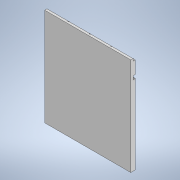
# Autodesk Inventor part: wall
Saved by Autodesk Inventor 2022 (Build 260153000, 153)
## iProperties
Created: 2022-02-20
Part Number: wall
Material: Generic
Document SubType Name: Modeling
Designer: MarkP
Density: 1 g/cm^3
Appearance: Default
Author: MarkP
Autodesk Inventor part; units mm, degrees
ref_plane "YZ Plane" through (0, 0, 0) normal (1, 0, 0) x (0, 1, 0)
ref_plane "XZ Plane" through (0, 0, 0) normal (0, 1, 0) x (-1, 0, 0)
ref_plane "XY Plane" through (0, 0, 0) normal (0, 0, 1) x (1, 0, 0)
sketch "Sketch1" plane through (0, 0, 0) normal (0, 0, 1) x (1, 0, 0)
  line L0 (0, 0) -> (750, 0)
  line L1 (750, 0) -> (750, 850)
  line L2 (750, 850) -> (0, 850)
  line L3 (0, 850) -> (0, 0)
  dimension "d0" = 750
  dimension "d1" = 850
  constraints: 8 end point, 2 parallel, 1 horizontal, 1 perpendicular
  measures "d0" distance of L2.end L1.end
  measures "d1" distance of L1.end L0.end
extrude "Extrusion1" add sketch "Sketch1" along normal blind 40
sketch "Sketch2" plane through (0, 850, 0) normal (0, 1, 0) x (1, 0, 0)
  line L0 (750, 0) -> (0, 0) projected
  line L1 (0, 0) -> (750, 0)
  line L2 (750, 0) -> (750, -20)
  line L3 (750, -20) -> (0, -20)
  line L4 (0, -20) -> (0, 0)
  dimension "d4" = 750
  dimension "d5" = 20
  constraints: 8 end point, 2 parallel, 1 horizontal, 1 perpendicular
  measures "d4" distance of L2.end L3.end
  measures "d5" distance of L1.end L2.end
extrude "Extrusion2" cut sketch "Sketch2" against normal blind 20
sketch "Sketch3" plane through (0, 850, 40) normal (0, 1, 0) x (1, 0, 0)
  line L0 (0, 20) -> (0, 0) projected
  circle A0 centre (562, 20) radius 5
  circle A1 centre (375, 20) radius 5
  circle A2 centre (188, 20) radius 5
  point P0 (0, 40)
  dimension "d11" = 10
  dimension "d12" = 10
  dimension "d13" = 10
  constraints: 3 centre point
  measures "d11" diameter of A0
  measures "d12" diameter of A1
  measures "d13" diameter of A2
extrude "Extrusion3" cut sketch "Sketch3" against normal blind 40
thread "Thread1" size "M10x1.5" class "6H" standard "ANSI Metric M Profile" full length
thread "Thread2" size "M10x1.5" class "6H" standard "ANSI Metric M Profile" full length
thread "Thread3" size "M10x1.5" class "6H" standard "ANSI Metric M Profile" full length
sketch "Sketch4" plane through (0, 0, 0) normal (0, 0, -1) x (-1, 0, 0)
  line L0 (-750, 720) -> (0, 720)
  line L1 (0, 850) -> (0, 0) projected
  line L2 (-750, 720) -> (0, 720)
  line L3 (0, 720) -> (0, 690)
  line L4 (0, 690) -> (-750, 690)
  line L5 (-750, 690) -> (-750, 720)
  line L6 (0, 690) -> (-420, 690)
  line L7 (-420, 690) -> (-420, 720)
  line L8 (-420, 720) -> (0, 720)
  line L9 (0, 720) -> (0, 690)
  dimension "d23" = 30
  dimension "d24" = 420
  dimension "d25" = 30
  constraints: 18 end point, 4 parallel, 2 horizontal, 2 perpendicular, 1 point on line
  measures "d23" distance of L2.end L3.end
  measures "d24" distance of L7.end L8.end
  measures "d25" distance of L6.end L7.end
extrude "Extrusion4" cut sketch "Sketch4" against normal blind 20 contours L0 L7 L4 L5
body "Solid1"
